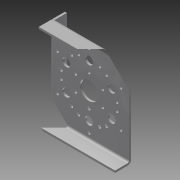
# Autodesk Inventor part: Plate 2 (Back)
Saved by Autodesk Inventor 2014 (Build 180170000, 170)
## iProperties
Created: 2014-01-12
Part Number: Plate 2 (Back)
Material: Steel
Document SubType Name: Sheet Metal
Designer: Andrew Toennies
Density: 7.85 g/cm^3
Sheet Metal Rule: Default
Appearance: Steel
Mass: 270.143 g
Surface Area: 251.295 cm^2
Volume: 34.4132 cm^3
Author: Andrew Toennies
Autodesk Inventor part; units mm, degrees
ref_plane "YZ Plane" through (0, 0, 0) normal (1, 0, 0) x (0, 1, 0)
ref_plane "XZ Plane" through (0, 0, 0) normal (0, 1, 0) x (-1, 0, 0)
ref_plane "XY Plane" through (0, 0, 0) normal (0, 0, 1) x (1, 0, 0)
sketch "Sketch1" plane through (0, 0, 0) normal (0, 0, 1) x (1, 0, 0)
  circle A0 centre (0, 0) radius 63.5 construction
  circle A1 centre (0, 0) radius 14.2875
  circle A2 centre (0, 41.275) radius 6.3881
  line L0 (0, 0) -> (0, 41.275) construction
  circle A3 centre (0, 41.275) radius 16.637 construction
  circle A4 centre (0, 57.912) radius 2.3812
  circle A5 centre (16.637, 41.275) radius 2.3812
  circle A6 centre (0, 24.638) radius 2.3812
  circle A7 centre (-16.637, 41.275) radius 2.3813
  line L1 (0, 41.275) -> (0, 57.912) construction
  line L2 (-16.637, 41.275) -> (16.637, 41.275) construction
  circle A8 centre (-50.1533, 28.956) radius 2.3812
  circle A9 centre (-44.0637, 6.2294) radius 2.3813
  circle A10 centre (-35.7452, 20.6375) radius 6.3881
  circle A11 centre (-27.4267, 35.0456) radius 2.3812
  circle A12 centre (-21.3371, 12.319) radius 2.3812
  circle A13 centre (-50.1533, -28.956) radius 2.3812
  circle A14 centre (-27.4267, -35.0456) radius 2.3813
  circle A15 centre (-35.7452, -20.6375) radius 6.3881
  circle A16 centre (-44.0637, -6.2294) radius 2.3812
  circle A17 centre (-21.3371, -12.319) radius 2.3812
  circle A18 centre (0, -57.912) radius 2.3812
  circle A19 centre (16.637, -41.275) radius 2.3813
  circle A20 centre (0, -41.275) radius 6.3881
  circle A21 centre (-16.637, -41.275) radius 2.3812
  circle A22 centre (0, -24.638) radius 2.3812
  circle A23 centre (50.1533, -28.956) radius 2.3812
  circle A24 centre (44.0637, -6.2294) radius 2.3813
  circle A25 centre (35.7452, -20.6375) radius 6.3881
  circle A26 centre (27.4267, -35.0456) radius 2.3812
  circle A27 centre (21.3371, -12.319) radius 2.3812
  circle A28 centre (50.1533, 28.956) radius 2.3812
  circle A29 centre (27.4267, 35.0456) radius 2.3813
  circle A30 centre (35.7452, 20.6375) radius 6.3881
  circle A31 centre (44.0637, 6.2294) radius 2.3812
  circle A32 centre (21.3371, 12.319) radius 2.3812
  line L3 (-63.5, 63.5) -> (63.5, 63.5)
  line L4 (63.5, 63.5) -> (63.5, -63.5)
  line L5 (63.5, -63.5) -> (-63.5, -63.5)
  line L6 (-63.5, -63.5) -> (-63.5, 63.5)
  dimension "d2" = 127
  dimension "d3" = 28.575
  dimension "d4" = 12.7762
  dimension "d5" = 41.275
  dimension "d6" = 33.274
  dimension "d7" = 4.7625
  dimension "d8" = 4.7625
  dimension "d9" = 4.7625
  dimension "d10" = 4.7625
  dimension "d11" = 360
  measures "d2" diameter of A0
  measures "d3" diameter of A1
  measures "d4" diameter of A2
  measures "d5" distance of L0.start L0.end
  measures "d6" diameter of A3
  measures "d7" diameter of A4
  measures "d8" diameter of A5
  measures "d9" diameter of A6
  measures "d10" diameter of A7
extrude "Plate1" add sketch "Sketch1" along normal blind 3.175
sketch "Sketch2" plane through (-60.325, 63.5, 3.175) normal (-1, 0, 0) x (0, -1, 0)
  line L0 (127, 0) -> (0, 0)
  line L1 (0, 0) -> (0, -25.4)
  line L2 (0, -25.4) -> (127, -25.4)
  line L3 (127, -25.4) -> (127, 0)
  constraints: 6 end point, 1 horizontal, 1 perpendicular, 1 vertical
edge flange "Flange1" height 25.4 angle 90 thickness 3.175 bend radius 3.175 thickness toward (-1, 0, 0) relief straight relief width 3.175 relief depth 1.5875 edges at (-63.5, 0, 0) wall of the first edge with corners at (-60.325, -63.5, 3.175) (-60.325, 63.5, 3.175) (-60.325, 63.5, -22.225) (-60.325, -63.5, -22.225)
bend "Bend1"
corner "Corner1"
sketch "Sketch3" plane through (63.5, -66.675, 6.35) normal (0, -1, 0) x (1, 0, 0)
  line L0 (-120.65, 0) -> (0, 0)
  line L1 (0, 0) -> (0, 19.05)
  line L2 (0, 19.05) -> (-120.65, 19.05)
  line L3 (-120.65, 19.05) -> (-120.65, 0)
  constraints: 6 end point, 1 horizontal, 1 perpendicular, 1 vertical
edge flange "Flange2" height 25.4 angle 90 thickness 3.175 bend radius 3.175 thickness toward (0, -1, 0) relief straight relief width 3.175 relief depth 1.5875 corner gap 3.175 corner form 0 edges at (3.175, -63.5, 3.175) (3.175, 63.5, 3.175) wall of the first edge with corners at (-57.15, -66.675, 6.35) (63.5, -66.675, 6.35) (63.5, -66.675, 25.4) (-57.15, -66.675, 25.4)
bend "Bend2"
corner "Corner2"
equation "\"d13\" = BendReliefWidth"
equation "\"d14\" = BendReliefDepth"
equation "\"d15\" = MinimumRemnant"
equation "\"d16\" = BendRadius"
equation "\"d20\" = CornerReliefSize"
equation "\"d21\" = GapSize"
equation "\"d22\" = JacobiRadiusSize"
equation "\"d23\" = BendReliefWidth"
equation "\"d24\" = BendReliefDepth"
equation "\"d25\" = MinimumRemnant"
equation "\"d26\" = BendRadius"
equation "\"d30\" = CornerReliefSize"
equation "\"d31\" = GapSize"
equation "\"d32\" = JacobiRadiusSize"
equation "\"BendRadius\" = Thickness"
equation "\"BendReliefWidth\" = Thickness"
equation "\"BendReliefDepth\" = 0.5 * Thickness"
equation "\"CornerReliefSize\" = 4 * Thickness"
equation "\"MinimumRemnant\" = 2 * Thickness"
equation "\"TransitionRadius\" = BendRadius"
equation "\"JacobiRadiusSize\" = BendRadius"
equation "\"GapSize\" = Thickness"
equation "\"d12\" = BendRadius"
equation "\"Thickness\" = 3.175"
body "Solid1"
